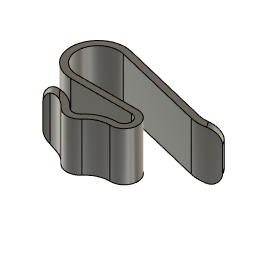
sunglass clip v2 (Autodesk Fusion 360 design; units mm, degrees)
Autodesk Fusion 360 part; units mm, degrees
sketch "Sketch1" plane through (0, 0, 0) normal (0, 0, 1) x (1, 0, 0)
  arc A0 (-47.973, 17) -> (-50, 0) centre (-50, 8.6208) ccw
  line L0 (-47.973, 17) -> (-11.0384, 8.0651)
  arc A1 (-11.0384, 8.0651) -> (0.1315, 9.8056) centre (-7.559, 22.4481) ccw
  line L1 (0.1315, 9.8056) -> (-1.3169, 11.9462)
  arc A2 (-10.4315, 10.5736) -> (-1.3169, 11.9462) centre (-7.559, 22.4481) ccw
  line L2 (-11.0384, 8.0651) -> (-10.4315, 10.5736)
  line L3 (-10.4315, 10.5736) -> (-47.3662, 19.5085)
  line L4 (-47.3662, 19.5085) -> (-47.973, 17)
  arc A3 (-47.3662, 19.5085) -> (-50, -2.5809) centre (-50, 8.6208) ccw
  line L5 (-50, 0) -> (-50, -2.5809)
  arc A4 (-50, -11.1599) -> (-52.2777, -11.8028) centre (-50, -15.5159) ccw
  arc A5 (-50, -8.5893) -> (-54.0306, -9.8827) centre (-50, -15.5159) ccw
  line L6 (-52.2777, -11.8028) -> (-54.0306, -9.8827)
  line L7 (-50, 0) -> (-48.5882, 0)
  line L8 (-48.5882, 0) -> (-25, 0)
  line L9 (-50, -2.5809) -> (-25, -2.5809)
  line L10 (-25, -2.5809) -> (-25, 0)
  line L11 (-50, -8.5893) -> (-25, -8.5893) construction
  line L12 (-50, -11.1599) -> (-25, -11.1599) construction
  line L13 (-25, -11.1599) -> (-25, -8.5893)
  line L14 (-25, -8.5893) -> (-25, -2.5809) construction
  arc A6 (-25, -8.5893) -> (-25, -2.5809) centre (-25, -5.5851) ccw
  arc A7 (-25.3384, -11.1599) -> (-25, 0) centre (-25, -5.5851) ccw
  arc A8 (-25.3384, -11.1599) -> (-33.1971, -14.8032) centre (-25.3384, -21.4571) ccw
  arc A9 (-41.7264, -14.8917) -> (-50, -11.1599) centre (-50, -22.1973) ccw
  arc A10 (-25, -8.5893) -> (-35.2112, -13.1865) centre (-25, -22.2281) ccw
  arc A11 (-39.7888, -13.1865) -> (-50, -8.5893) centre (-50, -22.2281) ccw
  arc A12 (-39.7888, -13.1865) -> (-35.2112, -13.1865) centre (-37.5, -11.1599) ccw
  arc A13 (-31.8618, -11.1599) -> (-31.9047, -10.4662) centre (-37.5, -11.1599) ccw
  arc A14 (-41.7264, -14.8917) -> (-33.1971, -14.8032) centre (-37.5, -11.1599) ccw
  dimension "d2" = 17
  dimension "d3" = 38
  dimension "d11" = 25
  dimension "d12" = 25
  dimension "d13" = 25
  dimension "d14" = 2.5808
  constraint tangent L0 A1
  constraint coincident A1.centre A2.centre
  constraint perpendicular L0 L2
  constraint tangent A2 L3
  constraint perpendicular L0 L4
  constraint coincident A0.centre A3.centre
  constraint coincident A4.centre A5.centre
  constraint tangent A0 L0
  constraint perpendicular L5 L8
  constraint tangent A3 L9
  constraint perpendicular L9 L10
  constraint horizontal L11
  constraint tangent A4 L12
  constraint parallel L9 L12
  constraint perpendicular L12 L13
  constraint midpoint L14 A6.centre
  constraint concentric A6 A7
  constraint vertical L14
  constraint coincident L12 A7.start
  constraint tangent L12 A8
  constraint tangent L12 A9
  constraint tangent L11 A10
  constraint tangent A10 A12
  constraint tangent A11 A12
  constraint tangent A5 A11
  constraint coincident A10 A13.end
  constraint coincident L12 A13.start
  measures "d2" vertical distance of A0.end A0.start
  measures "d3" distance of A0.start L0.end
  measures "d11" distance of A3.end L9.end
  measures "d12" distance of A5.start L11.end
  measures "d13" distance of A4.start L12.end
  measures "d14" distance of L8 L9
extrude "Extrude2" add sketch "Sketch1" along normal blind 20
fillet "Fillet3" radius 5 2 edges at (-0.5927, 10.8759, 20) (-0.5927, 10.8759, 0)
fillet "Fillet4" radius 5 2 edges at (-53.1541, -10.8428, 0) (-53.1541, -10.8428, 20)
sketch "Sketch2" plane through (1.8398, 7.6051, 0) normal (0.235129, 0.971964, 0) x (-0.971964, 0.235129, 0)
  line L0 (12.6252, 0) -> (50.6252, 0)
  line L1 (50.6252, 0) -> (50.6252, 20)
  line L2 (50.6252, 20) -> (12.6252, 20)
  line L3 (12.6252, 20) -> (12.6252, 0)
  line L4 (13.523, 1.3496) -> (30.9449, 1.3496) construction
  line L5 (30.9449, 1.3496) -> (30.9449, 6.3496) construction
  line L6 (30.9449, 6.3496) -> (13.523, 6.3496) construction
  line L7 (13.523, 6.3496) -> (13.523, 1.3496) construction
  text T0 "DroTron" font "Arial" height 5 align ink ink in box 0 x 0 at (13.523, 1.3496) x (1, 0) y (0, 1) spacing 1 kerned height is em
  constraint perpendicular L4 L5
  constraint parallel L4 L6
  constraint parallel L5 L7
extrude "Extrude3" cut sketch "Sketch2" against normal blind 0.5 text T0
extrude "Extrude1" [suppressed]
fillet "Fillet1" [suppressed]
fillet "Fillet2" [suppressed]
